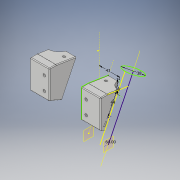
# Autodesk Inventor part: Marzocchi-380-Fix
Saved by Autodesk Inventor 2019.3 (Build 233278000, 278)
## iProperties
Created: 2019-01-16
Part Number: Marzocchi-380-Fix
Material: Generic
Document SubType Name: Modeling
Designer: eroldan
Density: 1 g/cm^3
Appearance: Default
Author: eroldan
Autodesk Inventor part; units mm, degrees
ref_plane "XZ Plane" through (0, 0, 0) normal (0, 1, 0) x (-1, 0, 0)
ref_plane "XY Plane" through (0, 0, 0) normal (0, 0, 1) x (1, 0, 0)
ref_plane "Work Plane2" through (72.5, 0, 0) normal (1, 0, 0) x (0, 1, 0)
sketch "Sketch2" plane through (72.5, 0, 0) normal (1, 0, 0) x (0, 1, 0)
  line L0 (0, 0) -> (0, 9.6252) construction
  line L1 (0, 0) -> (104.9991, -51.2115)
  dimension "headtube_angle" = 64
  constraints: 4 end point, 1 vertical
  measures "headtube_angle" angle of L0 L1
ref_plane "Work Plane3" through (72.5, 104.9991, -51.2115) normal (0, 0.898794, -0.4383711) x (-1, 0, 0)
sketch "Sketch3" plane through (72.5, 104.9991, -51.2115) normal (0, 0.898794, -0.4383711) x (-1, 0, 0)
  circle A0 centre (0, 0) radius 19
  point P0 (72.5, 0)
  dimension "diameter_stanchions" = 38
  constraints: 1 centre point
  measures "diameter_stanchions" diameter of A0
sweep "Sweep1" add profiles "Sketch3" path "Sketch2"
ref_plane "Work Plane4" through (32.5, 0, 0) normal (1, 0, 0) x (0, 1, 0)
sketch "Sketch4" plane through (32.5, 0, 0) normal (1, 0, 0) x (0, 1, 0)
  line L0 (0, 0) -> (104.9991, -51.2115) construction
  line L1 (83.3693, -40.6619) -> (21.2622, -10.3703)
  line L2 (21.2622, -10.3703) -> (31.9009, 15.5814)
  line L3 (31.9009, 15.5814) -> (90.0087, 15.5814)
  line L4 (90.0087, 1.6677) -> (83.3693, -40.6619)
  line L5 (83.3693, -40.6619) -> (90.0087, 1.6677)
  line L6 (90.0087, 15.5814) -> (90.0087, 1.6677)
  constraints: 12 end point, 2 point on line, 1 vertical
extrude "Extrusion1" add sketch "Sketch4" along normal up to surface (40 mm away) separate body
ref_plane "Work Plane5" through (32.5, 31.9009, -53.6686) normal (0, 0, 1) x (1, 0, 0)
sketch "Sketch6" plane through (32.5, 31.9009, -53.6686) normal (0, 0, 1) x (1, 0, 0)
  line L0 (-32.5, 105.7587) -> (-32.5, -64.5613) construction
  point P0 (-32.5, -31.9009)
  point P1 (10.5, 41.0717)
  point P2 (10.5, 13.0717)
  dimension "d11" = 28
  dimension "distance_lamp_holes" = 43
  constraints: 1 vertical alignment
  measures "d11" distance of point (10.5, 13.072) point (10.5, 41.072)
  measures "distance_lamp_holes" distance from line of L0 point (10.5, 41.072)
hole "Hole1" at (43, 72.9726, -53.6686) at (43, 44.9726, -53.6686) direction (0, 0, 1) diameter 5.5 end through all counterbore diameter 9.3 counterbore depth 54.75 bodies 2
sketch "Sketch11" plane through (72.5, 31.9009, 15.5814) normal (1, 0, 0) x (0, 0, -1)
  line L0 (-1.4957, -23.5718) -> (49.7158, 81.4273) projected
  line L1 (13.9137, 58.1079) -> (56.2433, 51.4685) projected
  line L2 (13.9137, 58.1079) -> (56.2433, 51.4685) projected
  point P0 (15.5814, -31.9009)
  point P1 (17.3178, 15.0016)
  point P2 (36.6062, 54.5486)
  dimension "d43" = 44
  constraints: 3 point on line
  measures "d43" distance of point (17.318, 15.002) point (36.606, 54.549)
sketch "Sketch12" plane through (72.5, 0, 0) normal (0, -0.898794, 0.4383711) x (1, 0, 0)
  circle A0 centre (0, 0) radius 18.125
  circle A1 centre (0, 0) radius 19 projected
  point P0 (-72.5, 0)
  dimension "d44" = 36.25
  constraints: 1 centre point
  measures "d44" diameter of A0
extrude "Extrusion2" cut sketch "Sketch12" against normal up to surface (42.9169 mm away) bodies 1
fillet "Fillet4" radius 1.75 1 edges at (54.375, 38.5734, -18.8135)
combine bodies "Combine1" operation type subtract main body 2 bodies to subtract 1 keep tools yes
sketch "Sketch9" plane through (72.5, 31.9009, 15.5814) normal (1, 0, 0) x (0, 0, -1)
  line L0 (-1.4957, -23.5718) -> (49.7158, 81.4273) construction
  line L1 (23.6956, 33.781) -> (27.4218, 41.4208)
  line L2 (27.4218, 41.4208) -> (24.995, 42.6044)
  line L3 (24.995, 42.6044) -> (21.2689, 34.9646)
  line L4 (21.2689, 34.9646) -> (23.6956, 33.781)
  line L5 (12.3025, 10.4215) -> (8.5763, 2.7818)
  line L6 (8.5763, 2.7818) -> (6.1496, 3.9654)
  line L7 (6.1496, 3.9654) -> (9.8757, 11.6051)
  line L8 (9.8757, 11.6051) -> (12.3025, 10.4215)
  line L9 (-3.6683, -71.3685) -> (86.1937, 112.8758) projected
  point P0 (15.5814, -31.9009)
  dimension "d27" = 8.5
  dimension "d28" = 2.7
  dimension "d29" = 2.5
  dimension "d30" = 8.5
  dimension "d33" = 2.5
  dimension "d34" = 2.7
  constraints: 16 end point, 5 perpendicular, 1 parallel
  measures "d27" distance of L1.start L1.end
  measures "d28" distance of L1.end L2.end
  measures "d29" distance between parallel lines of L0 L1
  measures "d30" distance of L5.start L5.end
  measures "d33" distance between parallel lines of L0 L5
  measures "d34" distance of L7.end L5.start
revolve "Revolution1" cut sketch "Sketch9" angle 360 about axis through (72.5, 0, 0) along (0, 0.898794, -0.4383711) bodies 2
fillet "Fillet3" radius 1.5 13 edges at (52.5, 90.0087, 15.5814) (72.5, 60.9548, 15.5814) (72.5, 90.0087, 8.6245) (52.5, 31.9009, 15.5814) (32.5, 60.9548, 15.5814) (32.5, 86.689, -19.4971) (32.5, 90.0087, 8.6245) (52.5, 90.0087, 1.6677) (72.5, 88.2291, -9.6785) (43, 83.3693, -40.6619) (32.5, 26.5816, 2.6056) (43.4375, 21.2622, -10.3703) (32.5, 52.3158, -25.5161)
sketch "Sketch10" plane through (34, 89.9906, 1.5522) normal (0, 0.9879214, -0.1549558) x (1, 0, 0)
  line L0 (0, 40.6999) -> (19.5994, 40.6999) projected
  line L1 (13.65, 39.3317) -> (13.65, 3.1021) construction
  line L2 (4.35, 39.3317) -> (4.35, 3.1021) construction
  line L3 (13.65, 39.3317) -> (13.65, 3.1021) construction
  line L4 (13.65, 23.526) -> (4.35, 23.526) construction
  point P0 (-34, 15.478)
  point P1 (9, 26.6999)
  point P2 (9, 23.526)
  dimension "d35" = 14
  constraints: 2 end point, 2 point on line, 1 midpoint, 1 perpendicular, 1 vertical alignment
  measures "d35" distance from line of point (9, 26.7) L0
hole "Hole2" at (43, 85.8533, -24.8252) direction (0, -0.9879214, 0.1549558) diameter 5.25 end up to face face through (43, 72.9726, -26.2936) facing (0, 0, 1) round with radius 4.65 far side no bodies 2
mirror "Mirror3" about plane through (0, 0, 0) normal (1, 0, 0) bodies 2 separate body
equation "\"d30\" = d27"
equation "\"d33\" = d29"
equation "\"d34\" = d28"
